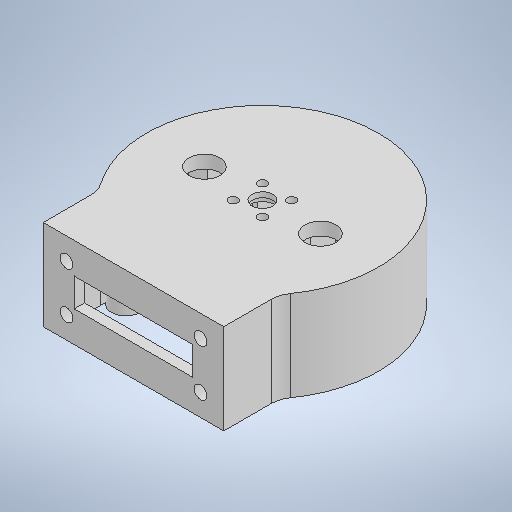
# Autodesk Inventor part: SCARA arm base
Saved by Autodesk Inventor 2025.2 (Build 292293000, 293)
## iProperties
Created: 2025-01-26
Part Number: SCARA arm base
Material: Generic
Document SubType Name: Modeling
Designer: caomi
Density: 1 g/cm^3
Appearance: Default
Author: caomi
Autodesk Inventor part; units mm, degrees
ref_plane "YZ Plane" through (0, 0, 0) normal (1, 0, 0) x (0, 1, 0)
ref_plane "XZ Plane" through (0, 0, 0) normal (0, 1, 0) x (-1, 0, 0)
ref_plane "XY Plane" through (0, 0, 0) normal (0, 0, 1) x (1, 0, 0)
sketch "Sketch1" plane through (0, 0, 0) normal (0, 1, 0) x (-1, 0, 0)
  circle A0 centre (0, 0) radius 45
  line L0 (89.3923, 0) -> (-44.3923, 0) construction
  line L1 (33.5, 5) -> (33.5, -5)
  line L2 (33.5, -5) -> (29.5, -8.3)
  line L3 (29.5, -8.3) -> (29.5, -15.35)
  line L4 (29.5, -15.35) -> (19.5, -15.35)
  line L5 (19.5, -15.35) -> (17.5, -17)
  line L6 (17.5, -17) -> (11.5, -17)
  line L7 (11.5, 17) -> (17.5, 17)
  line L8 (17.5, 17) -> (19.5, 15.35)
  line L9 (19.5, 15.35) -> (29.5, 15.35)
  line L10 (29.5, 15.35) -> (29.5, 8.3)
  line L11 (29.5, 8.3) -> (33.5, 5)
  line L12 (11.5, -17) -> (11.5, -7.25)
  line L13 (11.5, -7.25) -> (12.5, -6.25)
  line L14 (12.5, -6.25) -> (12.5, 6.25)
  line L15 (12.5, 6.25) -> (11.5, 7.25)
  line L16 (11.5, 7.25) -> (11.5, 17)
  circle A1 centre (22.5, 0) radius 6
  line L17 (13.233, 0) -> (-58.233, 0) construction
  line L18 (-33.5, -5) -> (-33.5, 5)
  line L19 (-33.5, 5) -> (-29.5, 8.3)
  line L20 (-29.5, 8.3) -> (-29.5, 15.35)
  line L21 (-29.5, 15.35) -> (-19.5, 15.35)
  line L22 (-19.5, 15.35) -> (-17.5, 17)
  line L23 (-17.5, 17) -> (-11.5, 17)
  line L24 (-11.5, -17) -> (-17.5, -17)
  line L25 (-17.5, -17) -> (-19.5, -15.35)
  line L26 (-19.5, -15.35) -> (-29.5, -15.35)
  line L27 (-29.5, -15.35) -> (-29.5, -8.3)
  line L28 (-29.5, -8.3) -> (-33.5, -5)
  line L29 (-11.5, 17) -> (-11.5, 7.25)
  line L30 (-11.5, 7.25) -> (-12.5, 6.25)
  line L31 (-12.5, 6.25) -> (-12.5, -6.25)
  line L32 (-12.5, -6.25) -> (-11.5, -7.25)
  line L33 (-11.5, -7.25) -> (-11.5, -17)
  circle A2 centre (-22.5, 0) radius 6
  line L34 (0, -29.964) -> (0, 34.746) construction
  line L35 (-35, 28.2843) -> (-35, 50)
  line L36 (-35, 50) -> (35, 50)
  line L37 (35, 50) -> (35, 28.2843)
  point P0 (11.5, -12.125)
  point P1 (-11.5, 12.125)
  dimension "d0" = 45
  dimension "d2" = 34
  dimension "d3" = 6
  dimension "d4" = 8
  dimension "d5" = 11
  dimension "d6" = 12
  dimension "d7" = 18
  dimension "d8" = 16.6
  dimension "d9" = 12.5
  dimension "d10" = 1
  dimension "d11" = 10
  dimension "d13" = 22
  dimension "d16" = 8
  dimension "d17" = 11
  dimension "d19" = 18
  dimension "d20" = 16.6
  dimension "d22" = 1
  dimension "d24" = 45
  dimension "d25" = 22
  dimension "d26" = 34
  dimension "d27" = 45
  dimension "d28" = 90
  dimension "d48" = 70
  dimension "d49" = 50
  constraints: 76 end point, 13 parallel, 6 midpoint, 6 perpendicular, 5 point on line, 4 vertical, 3 centre point, 2 collinear, 2 horizontal, 2 point on circle, 1 coincident, 1 equal radius, 16 other
  measures "d0" angle of L12 L13
  measures "d2" distance between parallel lines of L7 L6
  measures "d3" distance of L5.end L12.start
  measures "d4" distance from line of L12 L4.end
  measures "d5" distance from line of A1.centre L16
  measures "d6" diameter of A1
  measures "d7" distance between parallel lines of L12 L3
  measures "d8" distance of L2.end L11.start
  measures "d9" distance of L14.start L14.end
  measures "d10" distance between parallel lines of L14 L12
  measures "d11" distance of L1.start L1.end
  measures "d13" distance from line of point (-11.5, 12.125) L18
  measures "d16" distance from line of L29 L21.end
  measures "d17" distance from line of A2.centre L33
  measures "d19" distance between parallel lines of L29 L20
  measures "d20" distance of L19.end L28.start
  measures "d22" distance between parallel lines of L31 L29
  measures "d24" angle of L30 L29
  measures "d25" distance between parallel lines of L12 L1
  measures "d26" distance between parallel lines of L23 L24
  measures "d27" distance of A2.centre A1.centre
  measures "d28" diameter of A0
  measures "d48" distance of L35.end L36.end
  measures "d49" distance from line of L36 point (0, 0)
extrude "Extrusion1" add sketch "Sketch1" against normal blind 30 contours A0 | A0 L35 L36 L37
extrude "Extrusion2" add sketch "Sketch1" along normal blind 5 contours A0 | A0 L35 L36 L37 | L1 L2 L3 L4 L5 L6 L12 L13 L14 L15 L16 L7 L8 L9 L10 L11 | L18 L19 L20 L21 L22 L23 L29 L30 L31 L32 L33 L24 L25 L26 L27 L28
fillet "Fillet1" radius 10 2 edges at (-35, -12.5, 28.2843) (35, -12.5, 28.2843)
shell "Shell2" thickness 4 removed faces 1 at (-3.8333, -30, 39)
sketch "Sketch2" plane through (0, 1, 0) normal (0, -1, 0) x (-1, 0, 0)
  circle A0 centre (-5.6569, -5.6569) radius 1.75
  circle A1 centre (0, 0) radius 5
  circle A2 centre (0, 0) radius 4
  line L0 (-5.6569, -5.6569) -> (0, 0) construction
  line L1 (0, 0) -> (-7.2952, 0) construction
  dimension "d35" = 3.5
  dimension "d36" = 8
  dimension "d42" = 10
  dimension "d45" = 8
  dimension "d50" = 45
  constraints: 4 end point, 3 centre point, 2 coincident, 1 horizontal
  measures "d35" diameter of A0
  measures "d36" distance of point (0, 0) L0.start
  measures "d42" diameter of A1
  measures "d45" diameter of A2
  measures "d50" angle of L0 L1
extrude "Extrusion3" cut sketch "Sketch2" against normal blind 5 contours A0
pattern_circular "Circular Pattern1" count 4 over 360 about axis through (0, 0, 0) along (0, -1, 0) of "Extrusion3"
extrude "Extrusion4" cut sketch "Sketch2" against normal blind 2 contours A1 | A2
extrude "Extrusion5" cut sketch "Sketch2" against normal up to surface (4 mm away) contours A2
sketch "Sketch4" plane through (0, -30, 0) normal (0, -1, 0) x (1, 0, 0)
  line L0 (-26.5165, 26.5165) -> (0, 0) construction
  line L1 (0, 0) -> (-22.177, 0) construction
  circle A0 centre (-26.5165, 26.5165) radius 2.15
  line L2 (-24.1205, 30.6665) -> (-21.7245, 26.5165)
  line L3 (-21.7245, 26.5165) -> (-24.1205, 22.3665)
  line L4 (-24.1205, 22.3665) -> (-28.9125, 22.3665)
  line L5 (-28.9125, 22.3665) -> (-31.3085, 26.5165)
  line L6 (-31.3085, 26.5165) -> (-28.9125, 30.6665)
  line L7 (-28.9125, 30.6665) -> (-24.1205, 30.6665)
  circle A1 centre (-26.5165, 26.5165) radius 5.5
  line L8 (0, 0) -> (0, 20.5165) construction
  line L9 (-24.1205, 30.6665) -> (-22.9071, 30.6665)
  line L10 (-24.1205, 22.3665) -> (-22.9071, 22.3665)
  circle A2 centre (26.5165, 26.5165) radius 2.15
  line L11 (24.1205, 30.6665) -> (21.7245, 26.5165)
  line L12 (21.7245, 26.5165) -> (24.1205, 22.3665)
  line L13 (24.1205, 22.3665) -> (28.9125, 22.3665)
  line L14 (28.9125, 22.3665) -> (31.3085, 26.5165)
  line L15 (31.3085, 26.5165) -> (28.9125, 30.6665)
  line L16 (28.9125, 30.6665) -> (24.1205, 30.6665)
  circle A3 centre (26.5165, 26.5165) radius 5.5
  line L17 (24.1205, 30.6665) -> (22.9071, 30.6665)
  line L18 (24.1205, 22.3665) -> (22.9071, 22.3665)
  circle A4 centre (-26.5165, -26.5165) radius 2.15
  line L19 (-24.1205, -30.6665) -> (-21.7245, -26.5165)
  line L20 (-21.7245, -26.5165) -> (-24.1205, -22.3665)
  line L21 (-24.1205, -22.3665) -> (-28.9125, -22.3665)
  line L22 (-28.9125, -22.3665) -> (-31.3085, -26.5165)
  line L23 (-31.3085, -26.5165) -> (-28.9125, -30.6665)
  line L24 (-28.9125, -30.6665) -> (-24.1205, -30.6665)
  circle A5 centre (-26.5165, -26.5165) radius 5.5
  line L25 (-24.1205, -30.6665) -> (-22.9071, -30.6665)
  line L26 (-24.1205, -22.3665) -> (-22.9071, -22.3665)
  circle A6 centre (26.5165, -26.5165) radius 2.15
  line L27 (24.1205, -30.6665) -> (21.7245, -26.5165)
  line L28 (21.7245, -26.5165) -> (24.1205, -22.3665)
  line L29 (24.1205, -22.3665) -> (28.9125, -22.3665)
  line L30 (28.9125, -30.6665) -> (24.1205, -30.6665)
  line L31 (24.1205, -30.6665) -> (22.9071, -30.6665)
  line L32 (24.1205, -22.3665) -> (22.9071, -22.3665)
  circle A7 centre (26.5165, -26.5165) radius 5.5
  line L33 (28.9125, -22.3665) -> (31.3085, -26.5165)
  line L34 (31.3085, -26.5165) -> (28.9125, -30.6665)
  point P0 (0, -20.5165)
  dimension "d60" = 37.5
  dimension "d61" = 45
  dimension "d62" = 4.3
  dimension "d63" = 8.3
  dimension "d64" = 11
  constraints: 70 end point, 37 symmetric about line, 12 coincident, 8 centre point, 8 point on circle, 3 horizontal, 1 parallel, 1 vertical, 19 other
  measures "d60" distance of L0.start L0.end
  measures "d61" angle of L0 L1
  measures "d62" diameter of A0
  measures "d63" distance between parallel lines of L7 L4
  measures "d64" diameter of A1
extrude "Extrusion7" add sketch "Sketch4" against normal up to surface (31 mm away)
ref_plane "Work Plane1" through (0, -25, 0) normal (0, -1, 0) x (1, 0, 0)
extrude "Extrusion8" cut sketch "Sketch4" against normal blind 4.2 from surface at -5 contours L9 A1 L10 L3 L2 | L2 L3 L4 L5 L6 L7 | L16 L15 L14 L13 L12 L11 | L11 L12 L18 A3 L17 | L24 L23 L22 L21 L20 L19 | L19 L20 L26 A5 L25 | L31 A7 L32 L28 L27 | L27 L28 L29 L33 L34 L30
sketch "Sketch3" plane through (-35, -30, 50) normal (0, 0, 1) x (1, 0, 0)
  line L0 (70, 0) -> (70, 35) projected
  line L1 (70, 0) -> (0, 0) projected
  line L2 (0, 0) -> (0, 35) projected
  line L3 (0, 35) -> (70, 35) projected
  line L4 (12, 12) -> (58, 12)
  line L5 (58, 12) -> (58, 23)
  line L6 (58, 23) -> (12, 23)
  line L7 (12, 23) -> (12, 12)
  circle A0 centre (61, 8.5) radius 2.5
  circle A1 centre (61, 26.5) radius 2.5
  circle A2 centre (9, 26.5) radius 2.5
  circle A3 centre (9, 8.5) radius 2.5
  line L8 (35, -11.8491) -> (35, 83.4132) construction
  line L9 (47.5361, 17.5) -> (15.8673, 17.5) construction
  point P0 (0, 17.5)
  point P1 (35, 0)
  point P2 (12, 17.5)
  point P3 (35, 12)
  dimension "d51" = 12
  dimension "d54" = 5
  dimension "d56" = 52
  dimension "d57" = 18
  constraints: 12 end point, 4 centre point, 4 midpoint, 3 equal radius, 2 horizontal alignment, 2 point on line, 2 vertical alignment, 1 horizontal, 1 vertical, 5 other
  measures "d51" distance between parallel lines of L4 L1
  measures "d54" diameter of A0
  measures "d56" distance of A3.centre A0.centre
  measures "d57" distance of A1.centre A0.centre
extrude "Extrusion6" cut sketch "Sketch3" against normal up to surface (4 mm away) contours L7 L6 L5 L4 | A0 | A1 | A2 | A3
equation "\"d17\" = d5"
body "Solid1"
